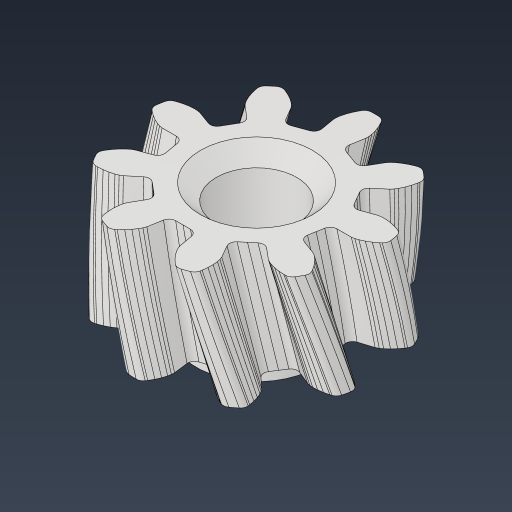
# Autodesk Inventor part: Planetengetriebe Planet
Saved by Autodesk Inventor 2023.1 (Build 271208000, 208)
## iProperties
Part Number: Planetengetriebe Planet
Material: Polyaryletherketon-Kunststoff
Document SubType Name: Modeling
Designer: rYan
Density: 1.32 g/cm^3
Appearance: Glatt - Weiß
Mass: 0.315298 g
Surface Area: 4.33242 cm^2
Volume: 0.238862 cm^3
Author: rYan
Autodesk Inventor part; units mm, degrees
ref_plane "YZ Plane" through (0, 0, 0) normal (1, 0, 0) x (0, 1, 0)
ref_plane "XZ Plane" through (0, 0, 0) normal (0, 1, 0) x (-1, 0, 0)
ref_plane "XY Plane" through (0, 0, 0) normal (0, 0, 1) x (1, 0, 0)
sketch "Skizze1" plane through (0, 0, 0) normal (0, 0, 1) x (1, 0, 0)
  circle A0 centre (0, 0) radius 3.3 construction
  circle A1 centre (0, 0) radius 4.2286 construction
  circle A2 centre (0, 0) radius 4.5 construction
  circle A3 centre (0, 0) radius 5.3 construction
  line L0 (0, 7.42) -> (0, -7.42) construction
  arc A4 (0.7096, 4.4437) -> (-0.7096, 4.4437) centre (0, 0) ccw
  arc A5 (0.729, 4.1653) -> (-0.729, 4.1653) centre (0, 0) ccw
  arc A6 (0.3429, 5.2889) -> (-0.3429, 5.2889) centre (0, 0) ccw
  line L1 (-0.729, 4.1653) -> (-0.6182, 3.5324)
  line L2 (0.729, 4.1653) -> (0.6182, 3.5324)
  arc A7 (0.6182, 3.5324) -> (0.8111, 3.1988) centre (0.9137, 3.4807) ccw
  arc A8 (-0.8111, 3.1988) -> (-0.6182, 3.5324) centre (-0.9137, 3.4807) ccw
  line L3 (0, 0) -> (1.1229, 3.0853)
  line L4 (0, 0) -> (-1.1229, 3.0853)
  line L5 (1.1229, 3.0853) -> (0.8111, 3.1988)
  line L6 (-0.8111, 3.1988) -> (-1.1229, 3.0853)
  arc A9 (0.5742, 4.8662) -> (-0.5742, 4.8662) centre (0, 0) ccw construction
  arc A10 (0.7294, 4.3029) -> (-0.7294, 4.3029) centre (0, 0) ccw construction
  arc A11 (0.4698, 5.0783) -> (-0.4698, 5.0783) centre (0, 0) ccw construction
  line L7 (0.3429, 5.2889) -> (0.4698, 5.0783)
  line L8 (0.4698, 5.0783) -> (0.5742, 4.8662)
  line L9 (0.7096, 4.4437) -> (0.7294, 4.3029)
  line L10 (0.7294, 4.3029) -> (0.729, 4.1653)
  arc A12 (0.655, 4.6541) -> (-0.655, 4.6541) centre (0, 0) ccw construction
  line L11 (0.5742, 4.8662) -> (0.655, 4.6541)
  line L12 (0.7096, 4.4437) -> (0.655, 4.6541)
  line L13 (-0.3429, 5.2889) -> (-0.4698, 5.0783)
  line L14 (-0.4698, 5.0783) -> (-0.5742, 4.8662)
  line L15 (-0.5742, 4.8662) -> (-0.655, 4.6541)
  line L16 (-0.655, 4.6541) -> (-0.7096, 4.4437)
  line L17 (-0.7096, 4.4437) -> (-0.7294, 4.3029)
  line L18 (-0.7294, 4.3029) -> (-0.729, 4.1653)
  dimension "d0" = 6.6
  dimension "d1" = 8.4572
  dimension "d2" = 9
  dimension "d3" = 10.6
  dimension "d4" = 1.4252
  dimension "d12" = 1.4653
  dimension "d13" = 0.6862
  dimension "d19" = 0.3
  dimension "d20" = 0.3
  dimension "d21" = 40
  dimension "d29" = 1.1511
  dimension "d30" = 4.9
  dimension "d31" = 4.3643
  dimension "d32" = 1.4657
  dimension "d33" = 5.1
  dimension "d34" = 0.9409
  dimension "d35" = 4.7
  dimension "d36" = 1.3142
  constraints: 36 end point, 26 point on circle, 13 centre point, 11 coincident, 7 symmetric about line, 4 tangent, 2 perpendicular, 2 point on line, 1 other
  measures "d0" diameter of A0
  measures "d1" diameter of A1
  measures "d2" diameter of A2
  measures "d3" diameter of A3
  measures "d19" radius of A7
  measures "d20" radius of A8
  measures "d21" angle of L3 L4
  measures "d30" radius of A9
  measures "d31" radius of A10
  measures "d33" radius of A11
  measures "d35" radius of A12
coil "Spirale2" sketch "Skizze1" operation add axis through (0, 0, -10) along (0, 0, -1) pitch 104.0668 turns 0.048046 hand left
fillet "Rundung2" radius 0.3 2 edges at (-1.1343, 5.1772, -2.5) (-0.4563, 5.2803, -2.5)
pattern_circular "Runde Anordnung4" count 9 over 360 about axis through (0, 0, -10) along (0, 0, 1) of "Spirale2", "Rundung2"
sketch "Skizze2" plane through (0, 0, 0) normal (0, 0, 1) x (1, 0, 0)
  point P0 (0, 0)
  point P1 (0, 0)
  constraints: 1 coincident
hole "Bohrung1" at (0, 0, 0) direction (0, 0, -1) diameter 3.6 end through all
sketch "Skizze4" plane through (-0.1031, 0.7973, -5) normal (0, 0, -1) x (-0.7537864, -0.6571196, 0)
  circle A0 centre (0.4462, -0.6688) radius 2.7
  circle A1 centre (0.4462, -0.6688) radius 1.8 projected
  dimension "d40" = 5.4
  constraints: 2 coincident, 1 centre point
  measures "d40" diameter of A0
extrude "Extrusion3" add sketch "Skizze4" along normal blind 0.8
chamfer "Fase1" distance 0.5 angle 45 1 edges at (1.3568, 1.1828, -5.8)
chamfer "Fase2" distance 0.7 angle 45 1 edges at (0, 1.8, 0)
sketch "Skizze10" plane through (-0.6182, 3.5324, 0) normal (0, 0, 1) x (0.9850278, 0.1723953, 0)
  arc A0 (1.0773, 1.6033) -> (0.7491, 1.6607) centre (0, -3.5861) ccw projected
  line L0 (0.4653, 1.5576) -> (0.4127, 1.4972) projected
  line L1 (0.4127, 1.4972) -> (0.2733, 1.3063) projected
  line L2 (0.2733, 1.3063) -> (0.1572, 1.1113) projected
  line L3 (0.1572, 1.1113) -> (0.0671, 0.9134) projected
  line L4 (0.0671, 0.9134) -> (0.0233, 0.7782) projected
  line L5 (0.0233, 0.7782) -> (0, 0.6425) projected
  line L6 (0, 0.6425) -> (0, 0) projected
  arc A1 (-0.2475, -0.2954) -> (0, 0) centre (-0.3, 0) ccw projected
  line L7 (-0.2475, -0.2954) -> (-0.5742, -0.3534) projected
  line L8 (-0.5742, -0.3534) -> (-0.901, -0.4115) projected
  arc A2 (-1.2351, -0.2194) -> (-0.901, -0.4115) centre (-0.9534, -0.1161) ccw projected
  line L9 (-1.2351, -0.2194) -> (-1.4564, 0.3838) projected
  line L10 (-1.4564, 0.3838) -> (-1.525, 0.5031) projected
  line L11 (-1.525, 0.5031) -> (-1.6126, 0.615) projected
  line L12 (-1.6126, 0.615) -> (-1.7654, 0.7698) projected
  line L13 (-1.7654, 0.7698) -> (-1.9415, 0.9129) projected
  line L14 (-1.9415, 0.9129) -> (-2.1382, 1.0441) projected
  line L15 (-2.1382, 1.0441) -> (-2.2084, 1.0827) projected
  arc A3 (-2.5104, 1.0817) -> (-2.7987, 0.9147) centre (0, -3.5861) ccw projected
  line L16 (-2.9499, 0.6533) -> (-2.9513, 0.5732) projected
  line L17 (-2.9513, 0.5732) -> (-2.9354, 0.3373) projected
  line L18 (-2.9354, 0.3373) -> (-2.899, 0.1134) projected
  line L19 (-2.899, 0.1134) -> (-2.8408, -0.0962) projected
  line L20 (-2.8408, -0.0962) -> (-2.7874, -0.2279) projected
  line L21 (-2.7874, -0.2279) -> (-2.7181, -0.3468) projected
  line L22 (-2.7181, -0.3468) -> (-2.3051, -0.839) projected
  arc A4 (-2.3048, -1.2244) -> (-2.3051, -0.839) centre (-2.5349, -1.0318) ccw projected
  line L23 (-2.3048, -1.2244) -> (-2.5178, -1.4788) projected
  line L24 (-2.5178, -1.4788) -> (-2.7308, -1.7333) projected
  arc A5 (-3.1102, -1.8009) -> (-2.7308, -1.7333) centre (-2.9608, -1.5408) ccw projected
  line L25 (-3.1102, -1.8009) -> (-3.6675, -1.4811) projected
  line L26 (-3.6675, -1.4811) -> (-3.7967, -1.4338) projected
  line L27 (-3.7967, -1.4338) -> (-3.9358, -1.4044) projected
  line L28 (-3.9358, -1.4044) -> (-4.1523, -1.3841) projected
  line L29 (-4.1523, -1.3841) -> (-4.3792, -1.3877) projected
  line L30 (-4.3792, -1.3877) -> (-4.6141, -1.4136) projected
  line L31 (-4.6141, -1.4136) -> (-4.6927, -1.4291) projected
  arc A6 (-4.9234, -1.624) -> (-5.037, -1.9372) centre (0, -3.5861) ccw projected
  line L32 (-4.9848, -2.2347) -> (-4.9344, -2.2969) projected
  line L33 (-4.9344, -2.2969) -> (-4.7706, -2.4674) projected
  line L34 (-4.7706, -2.4674) -> (-4.5987, -2.6156) projected
  line L35 (-4.5987, -2.6156) -> (-4.4195, -2.7387) projected
  line L36 (-4.4195, -2.7387) -> (-4.2939, -2.8053) projected
  line L37 (-4.2939, -2.8053) -> (-4.1644, -2.8518) projected
  line L38 (-4.1644, -2.8518) -> (-3.5316, -2.9634) projected
  arc A7 (-3.2837, -3.2584) -> (-3.5316, -2.9634) centre (-3.5837, -3.2588) ccw projected
  line L39 (-3.2837, -3.2584) -> (-3.2833, -3.5903) projected
  line L40 (-3.2833, -3.5903) -> (-3.2828, -3.9221) projected
  arc A8 (-3.53, -4.2178) -> (-3.2828, -3.9221) centre (-3.5828, -3.9225) ccw projected
  line L41 (-3.53, -4.2178) -> (-4.1625, -4.331) projected
  line L42 (-4.1625, -4.331) -> (-4.2919, -4.3778) projected
  line L43 (-4.2919, -4.3778) -> (-4.4173, -4.4447) projected
  line L44 (-4.4173, -4.4447) -> (-4.5962, -4.5683) projected
  line L45 (-4.5962, -4.5683) -> (-4.7677, -4.7169) projected
  line L46 (-4.7677, -4.7169) -> (-4.9311, -4.8878) projected
  line L47 (-4.9311, -4.8878) -> (-4.9813, -4.9502) projected
  arc A9 (-5.0328, -5.2478) -> (-4.9184, -5.5607) centre (0, -3.5861) ccw projected
  line L48 (-4.6872, -5.755) -> (-4.6086, -5.7703) projected
  line L49 (-4.6086, -5.7703) -> (-4.3736, -5.7956) projected
  line L50 (-4.3736, -5.7956) -> (-4.1466, -5.7986) projected
  line L51 (-4.1466, -5.7986) -> (-3.9302, -5.7777) projected
  line L52 (-3.9302, -5.7777) -> (-3.7912, -5.748) projected
  line L53 (-3.7912, -5.748) -> (-3.6621, -5.7004) projected
  line L54 (-3.6621, -5.7004) -> (-3.1056, -5.3791) projected
  arc A10 (-2.7261, -5.4458) -> (-3.1056, -5.3791) centre (-2.9556, -5.6389) ccw projected
  line L55 (-2.7261, -5.4458) -> (-2.5124, -5.6997) projected
  line L56 (-2.5124, -5.6997) -> (-2.2988, -5.9537) projected
  arc A11 (-2.2981, -6.339) -> (-2.2988, -5.9537) centre (-2.5284, -6.1468) ccw projected
  line L57 (-2.2981, -6.339) -> (-2.7099, -6.8323) projected
  line L58 (-2.7099, -6.8323) -> (-2.7789, -6.9514) projected
  line L59 (-2.7789, -6.9514) -> (-2.832, -7.0832) projected
  line L60 (-2.832, -7.0832) -> (-2.8896, -7.2929) projected
  line L61 (-2.8896, -7.2929) -> (-2.9254, -7.517) projected
  line L62 (-2.9254, -7.517) -> (-2.9407, -7.7529) projected
  line L63 (-2.9407, -7.7529) -> (-2.9391, -7.833) projected
  arc A12 (-2.7872, -8.094) -> (-2.4985, -8.2602) centre (0, -3.5861) ccw projected
  line L64 (-2.1965, -8.2605) -> (-2.1264, -8.2216) projected
  line L65 (-2.1264, -8.2216) -> (-1.9301, -8.0899) projected
  line L66 (-1.9301, -8.0899) -> (-1.7543, -7.9464) projected
  line L67 (-1.7543, -7.9464) -> (-1.6019, -7.7913) projected
  line L68 (-1.6019, -7.7913) -> (-1.5146, -7.6792) projected
  line L69 (-1.5146, -7.6792) -> (-1.4463, -7.5597) projected
  line L70 (-1.4463, -7.5597) -> (-1.2265, -6.9559) projected
  arc A13 (-0.8929, -6.763) -> (-1.2265, -6.9559) centre (-0.9446, -7.0585) ccw projected
  line L71 (-0.8929, -6.763) -> (-0.566, -6.8202) projected
  line L72 (-0.566, -6.8202) -> (-0.2392, -6.8774) projected
  arc A14 (0.0091, -7.1721) -> (-0.2392, -6.8774) centre (-0.2909, -7.1729) ccw projected
  line L73 (0.0091, -7.1721) -> (0.0108, -7.8147) projected
  line L74 (0.0108, -7.8147) -> (0.0344, -7.9503) projected
  line L75 (0.0344, -7.9503) -> (0.0785, -8.0854) projected
  line L76 (0.0785, -8.0854) -> (0.1692, -8.283) projected
  line L77 (0.1692, -8.283) -> (0.2857, -8.4777) projected
  line L78 (0.2857, -8.4777) -> (0.4256, -8.6683) projected
  line L79 (0.4256, -8.6683) -> (0.4784, -8.7286) projected
  arc A15 (0.7625, -8.8309) -> (1.0905, -8.7727) centre (0, -3.5861) ccw projected
  line L80 (1.322, -8.5787) -> (1.3508, -8.504) projected
  line L81 (1.3508, -8.504) -> (1.4165, -8.2769) projected
  line L82 (1.4165, -8.2769) -> (1.4589, -8.0539) projected
  line L83 (1.4589, -8.0539) -> (1.4759, -7.8372) projected
  line L84 (1.4759, -7.8372) -> (1.4707, -7.6951) projected
  line L85 (1.4707, -7.6951) -> (1.4463, -7.5597) projected
  line L86 (1.4463, -7.5597) -> (1.2265, -6.9559) projected
  arc A16 (1.3581, -6.5937) -> (1.2265, -6.9559) centre (1.5084, -6.8533) ccw projected
  line L87 (1.3581, -6.5937) -> (1.6453, -6.4274) projected
  line L88 (1.6453, -6.4274) -> (1.9324, -6.2611) projected
  arc A17 (2.3121, -6.3273) -> (1.9324, -6.2611) centre (2.0827, -6.5207) ccw projected
  line L89 (2.3121, -6.3273) -> (2.7263, -6.8185) projected
  line L90 (2.7263, -6.8185) -> (2.8316, -6.9071) projected
  line L91 (2.8316, -6.9071) -> (2.9522, -6.9823) projected
  line L92 (2.9522, -6.9823) -> (3.1487, -7.0754) projected
  line L93 (3.1487, -7.0754) -> (3.3632, -7.1497) projected
  line L94 (3.3632, -7.1497) -> (3.5928, -7.2057) projected
  line L95 (3.5928, -7.2057) -> (3.672, -7.218) projected
  arc A18 (3.9554, -7.1138) -> (4.1693, -6.8583) centre (0, -3.5861) ccw projected
  line L96 (4.222, -6.5609) -> (4.1959, -6.4851) projected
  line L97 (4.1959, -6.4851) -> (4.1003, -6.2689) projected
  line L98 (4.1003, -6.2689) -> (3.9894, -6.0709) projected
  line L99 (3.9894, -6.0709) -> (3.8631, -5.8939) projected
  line L100 (3.8631, -5.8939) -> (3.7679, -5.7884) projected
  line L101 (3.7679, -5.7884) -> (3.6621, -5.7004) projected
  line L102 (3.6621, -5.7004) -> (3.1056, -5.3791) projected
  arc A19 (2.9736, -5.0171) -> (3.1056, -5.3791) centre (3.2556, -5.1193) ccw projected
  line L103 (2.9736, -5.0171) -> (3.0867, -4.7051) projected
  line L104 (3.0867, -4.7051) -> (3.1998, -4.3931) projected
  arc A20 (3.5332, -4.1998) -> (3.1998, -4.3931) centre (3.4818, -4.4954) ccw projected
  line L105 (3.5332, -4.1998) -> (4.1662, -4.3098) projected
  line L106 (4.1662, -4.3098) -> (4.3038, -4.31) projected
  line L107 (4.3038, -4.31) -> (4.4446, -4.2901) projected
  line L108 (4.4446, -4.2901) -> (4.655, -4.2351) projected
  line L109 (4.655, -4.2351) -> (4.867, -4.1541) projected
  line L110 (4.867, -4.1541) -> (5.0789, -4.0494) projected
  line L111 (5.0789, -4.0494) -> (5.1475, -4.008) projected
  arc A21 (5.2976, -3.7459) -> (5.2972, -3.4128) centre (0, -3.5861) ccw projected
  line L112 (5.1464, -3.1511) -> (5.0777, -3.1098) projected
  line L113 (5.0777, -3.1098) -> (4.8655, -3.0056) projected
  line L114 (4.8655, -3.0056) -> (4.6533, -2.9252) projected
  line L115 (4.6533, -2.9252) -> (4.4428, -2.8708) projected
  line L116 (4.4428, -2.8708) -> (4.302, -2.8512) projected
  line L117 (4.302, -2.8512) -> (4.1644, -2.8518) projected
  line L118 (4.1644, -2.8518) -> (3.5316, -2.9634) projected
  arc A22 (3.1977, -2.7709) -> (3.5316, -2.9634) centre (3.4795, -2.6679) ccw projected
  line L119 (3.1977, -2.7709) -> (3.0838, -2.4592) projected
  line L120 (3.0838, -2.4592) -> (2.9699, -2.1475) projected
  arc A23 (3.1011, -1.7851) -> (2.9699, -2.1475) centre (3.2517, -2.0446) ccw projected
  line L121 (3.1011, -1.7851) -> (3.6567, -1.4625) projected
  line L122 (3.6567, -1.4625) -> (3.7623, -1.3742) projected
  line L123 (3.7623, -1.3742) -> (3.8573, -1.2684) projected
  line L124 (3.8573, -1.2684) -> (3.9831, -1.0911) projected
  line L125 (3.9831, -1.0911) -> (4.0934, -0.8928) projected
  line L126 (4.0934, -0.8928) -> (4.1885, -0.6764) projected
  line L127 (4.1885, -0.6764) -> (4.2144, -0.6005) projected
  arc A24 (4.1609, -0.3033) -> (3.9465, -0.0483) centre (0, -3.5861) ccw projected
  line L128 (3.6627, 0.0552) -> (3.5836, 0.0426) projected
  line L129 (3.5836, 0.0426) -> (3.3541, -0.014) projected
  line L130 (3.3541, -0.014) -> (3.1398, -0.0887) projected
  line L131 (3.1398, -0.0887) -> (2.9436, -0.1824) projected
  line L132 (2.9436, -0.1824) -> (2.8231, -0.2579) projected
  line L133 (2.8231, -0.2579) -> (2.7181, -0.3468) projected
  line L134 (2.7181, -0.3468) -> (2.3051, -0.839) projected
  arc A25 (1.9256, -0.9061) -> (2.3051, -0.839) centre (2.0753, -0.6461) ccw projected
  line L135 (1.9256, -0.9061) -> (1.638, -0.7406) projected
  line L136 (1.638, -0.7406) -> (1.3504, -0.575) projected
  arc A26 (1.2179, -0.2132) -> (1.3504, -0.575) centre (1.5001, -0.315) ccw projected
  line L137 (1.2179, -0.2132) -> (1.4362, 0.3912) projected
  line L138 (1.4362, 0.3912) -> (1.4603, 0.5267) projected
  line L139 (1.4603, 0.5267) -> (1.4651, 0.6687) projected
  line L140 (1.4651, 0.6687) -> (1.4475, 0.8855) projected
  line L141 (1.4475, 0.8855) -> (1.4046, 1.1083) projected
  line L142 (1.4046, 1.1083) -> (1.3382, 1.3352) projected
  line L143 (1.3382, 1.3352) -> (1.3093, 1.4099) projected
  circle A27 centre (0, -3.5861) radius 2.5 projected
  line L144 (3.632, -7.0094) -> (3.4197, -6.9576)
  line L145 (3.4197, -6.9576) -> (3.2245, -6.89)
  line L146 (3.2245, -6.89) -> (3.0483, -6.8065)
  line L147 (3.0483, -6.8065) -> (2.9495, -6.7449)
  line L148 (2.9495, -6.7449) -> (2.8682, -6.6765)
  line L149 (2.8682, -6.6765) -> (2.465, -6.1984)
  arc A28 (2.465, -6.1984) -> (1.8322, -6.088) centre (2.0827, -6.5207) ccw
  line L150 (1.8322, -6.088) -> (1.545, -6.2543)
  line L151 (1.545, -6.2543) -> (1.2579, -6.4206)
  arc A29 (1.2579, -6.4206) -> (1.0386, -7.0243) centre (1.5084, -6.8533) ccw
  line L152 (1.0386, -7.0243) -> (1.2525, -7.612)
  line L153 (1.2525, -7.612) -> (1.2714, -7.7166)
  line L154 (1.2714, -7.7166) -> (1.2756, -7.8329)
  line L155 (1.2756, -7.8329) -> (1.2603, -8.0274)
  line L156 (1.2603, -8.0274) -> (1.2218, -8.2303)
  line L157 (1.2218, -8.2303) -> (1.161, -8.4402)
  line L158 (1.161, -8.4402) -> (1.1353, -8.507)
  arc A30 (0.7337, -8.633) -> (1.0494, -8.5769) centre (0, -3.5861) ccw
  line L159 (0.629, -8.597) -> (0.5818, -8.5431)
  line L160 (0.5818, -8.5431) -> (0.4525, -8.3669)
  line L161 (0.4525, -8.3669) -> (0.3464, -8.1897)
  line L162 (0.3464, -8.1897) -> (0.2651, -8.0125)
  line L163 (0.2651, -8.0125) -> (0.229, -7.9018)
  line L164 (0.229, -7.9018) -> (0.2107, -7.7971)
  line L165 (0.2107, -7.7971) -> (0.2091, -7.1716)
  arc A31 (0.2091, -7.1716) -> (-0.2047, -6.6804) centre (-0.2909, -7.1729) ccw
  line L166 (-0.2047, -6.6804) -> (-0.5315, -6.6232)
  line L167 (-0.5315, -6.6232) -> (-0.8584, -6.566)
  arc A32 (-0.8584, -6.566) -> (-1.4144, -6.8875) centre (-0.9446, -7.0585) ccw
  line L168 (-1.4144, -6.8875) -> (-1.6284, -7.4752)
  line L169 (-1.6284, -7.4752) -> (-1.6811, -7.5675)
  line L170 (-1.6811, -7.5675) -> (-1.7527, -7.6593)
  line L171 (-1.7527, -7.6593) -> (-1.8893, -7.7984)
  line L172 (-1.8893, -7.7984) -> (-2.0493, -7.9291)
  line L173 (-2.0493, -7.9291) -> (-2.2308, -8.0508)
  line L174 (-2.2308, -8.0508) -> (-2.2934, -8.0855)
  arc A33 (-2.6821, -7.9239) -> (-2.4042, -8.0838) centre (0, -3.5861) ccw
  line L175 (-2.7391, -7.8289) -> (-2.7406, -7.7573)
  line L176 (-2.7406, -7.7573) -> (-2.7265, -7.5393)
  line L177 (-2.7265, -7.5393) -> (-2.6938, -7.3353)
  line L178 (-2.6938, -7.3353) -> (-2.6421, -7.1473)
  line L179 (-2.6421, -7.1473) -> (-2.5987, -7.0393)
  line L180 (-2.5987, -7.0393) -> (-2.5454, -6.9474)
  line L181 (-2.5454, -6.9474) -> (-2.1446, -6.4672)
  arc A34 (-2.1446, -6.4672) -> (-2.1458, -5.8249) centre (-2.5284, -6.1468) ccw
  line L182 (-2.1458, -5.8249) -> (-2.3594, -5.571)
  line L183 (-2.3594, -5.571) -> (-2.573, -5.317)
  arc A35 (-2.573, -5.317) -> (-3.2056, -5.2059) centre (-2.9556, -5.6389) ccw
  line L184 (-3.2056, -5.2059) -> (-3.7473, -5.5186)
  line L185 (-3.7473, -5.5186) -> (-3.847, -5.5554)
  line L186 (-3.847, -5.5554) -> (-3.9608, -5.5798)
  line L187 (-3.9608, -5.5798) -> (-4.1549, -5.5985)
  line L188 (-4.1549, -5.5985) -> (-4.3615, -5.5958)
  line L189 (-4.3615, -5.5958) -> (-4.5787, -5.5724)
  line L190 (-4.5787, -5.5724) -> (-4.6491, -5.5587)
  arc A36 (-4.8429, -5.185) -> (-4.7328, -5.4862) centre (0, -3.5861) ccw
  line L191 (-4.8256, -5.0756) -> (-4.7806, -5.0198)
  line L192 (-4.7806, -5.0198) -> (-4.6297, -4.8619)
  line L193 (-4.6297, -4.8619) -> (-4.4735, -4.7266)
  line L194 (-4.4735, -4.7266) -> (-4.3131, -4.6158)
  line L195 (-4.3131, -4.6158) -> (-4.2104, -4.561)
  line L196 (-4.2104, -4.561) -> (-4.1105, -4.5248)
  line L197 (-4.1105, -4.5248) -> (-3.4948, -4.4147)
  arc A37 (-3.4948, -4.4147) -> (-3.0828, -3.9218) centre (-3.5828, -3.9225) ccw
  line L198 (-3.0828, -3.9218) -> (-3.0833, -3.59)
  line L199 (-3.0833, -3.59) -> (-3.0837, -3.2582)
  arc A38 (-3.0837, -3.2582) -> (-3.4969, -2.7664) centre (-3.5837, -3.2588) ccw
  line L200 (-3.4969, -2.7664) -> (-4.1128, -2.6578)
  line L201 (-4.1128, -2.6578) -> (-4.2129, -2.6219)
  line L202 (-4.2129, -2.6219) -> (-4.3157, -2.5674)
  line L203 (-4.3157, -2.5674) -> (-4.4764, -2.4569)
  line L204 (-4.4764, -2.4569) -> (-4.6329, -2.3221)
  line L205 (-4.6329, -2.3221) -> (-4.7843, -2.1645)
  line L206 (-4.7843, -2.1645) -> (-4.8293, -2.1088)
  arc A39 (-4.7376, -1.698) -> (-4.8469, -1.9994) centre (0, -3.5861) ccw
  line L207 (-4.6541, -1.6253) -> (-4.5838, -1.6115)
  line L208 (-4.5838, -1.6115) -> (-4.3666, -1.5875)
  line L209 (-4.3666, -1.5875) -> (-4.16, -1.5842)
  line L210 (-4.16, -1.5842) -> (-3.9659, -1.6025)
  line L211 (-3.9659, -1.6025) -> (-3.852, -1.6265)
  line L212 (-3.852, -1.6265) -> (-3.7522, -1.663)
  line L213 (-3.7522, -1.663) -> (-3.2097, -1.9744)
  arc A40 (-3.2097, -1.9744) -> (-2.5774, -1.8617) centre (-2.9608, -1.5408) ccw
  line L214 (-2.5774, -1.8617) -> (-2.3644, -1.6072)
  line L215 (-2.3644, -1.6072) -> (-2.1515, -1.3527)
  arc A41 (-2.1515, -1.3527) -> (-2.1519, -0.7104) centre (-2.5349, -1.0318) ccw
  line L216 (-2.1519, -0.7104) -> (-2.5539, -0.2313)
  line L217 (-2.5539, -0.2313) -> (-2.6075, -0.1395)
  line L218 (-2.6075, -0.1395) -> (-2.6512, -0.0316)
  line L219 (-2.6512, -0.0316) -> (-2.7033, 0.1563)
  line L220 (-2.7033, 0.1563) -> (-2.7365, 0.3602)
  line L221 (-2.7365, 0.3602) -> (-2.7512, 0.5782)
  line L222 (-2.7512, 0.5782) -> (-2.7499, 0.6498)
  arc A42 (-2.4156, 0.9056) -> (-2.6931, 0.7449) centre (0, -3.5861) ccw
  line L223 (-2.3049, 0.9075) -> (-2.2421, 0.873)
  line L224 (-2.2421, 0.873) -> (-2.0603, 0.7517)
  line L225 (-2.0603, 0.7517) -> (-1.9, 0.6214)
  line L226 (-1.9, 0.6214) -> (-1.763, 0.4827)
  line L227 (-1.763, 0.4827) -> (-1.6912, 0.391)
  line L228 (-1.6912, 0.391) -> (-1.6383, 0.2989)
  line L229 (-1.6383, 0.2989) -> (-1.4228, -0.2883)
  arc A43 (-1.4228, -0.2883) -> (-0.866, -0.6084) centre (-0.9534, -0.1161) ccw
  line L230 (-0.866, -0.6084) -> (-0.5393, -0.5503)
  line L231 (-0.5393, -0.5503) -> (-0.2125, -0.4923)
  arc A44 (-0.2125, -0.4923) -> (0.2, 0) centre (-0.3, 0) ccw
  line L232 (0.2, 0) -> (0.2, 0.6255)
  line L233 (0.2, 0.6255) -> (0.218, 0.7302)
  line L234 (0.218, 0.7302) -> (0.2538, 0.841)
  line L235 (0.2538, 0.841) -> (0.3347, 1.0184)
  line L236 (0.3347, 1.0184) -> (0.4403, 1.1959)
  line L237 (0.4403, 1.1959) -> (0.5692, 1.3724)
  line L238 (0.5692, 1.3724) -> (0.6162, 1.4264)
  arc A45 (1.0367, 1.4074) -> (0.7209, 1.4627) centre (0, -3.5861) ccw
  line L239 (1.1228, 1.3378) -> (1.1487, 1.271)
  line L240 (1.1487, 1.271) -> (1.21, 1.0612)
  line L241 (1.21, 1.0612) -> (1.249, 0.8584)
  line L242 (1.249, 0.8584) -> (1.2648, 0.664)
  line L243 (1.2648, 0.664) -> (1.2609, 0.5477)
  line L244 (1.2609, 0.5477) -> (1.2422, 0.4431)
  line L245 (1.2422, 0.4431) -> (1.0298, -0.1452)
  arc A46 (1.0298, -0.1452) -> (1.2507, -0.7484) centre (1.5001, -0.315) ccw
  line L246 (1.2507, -0.7484) -> (1.5382, -0.9139)
  line L247 (1.5382, -0.9139) -> (1.8258, -1.0795)
  arc A47 (1.8258, -1.0795) -> (2.4583, -0.9675) centre (2.0753, -0.6461) ccw
  line L248 (2.4583, -0.9675) -> (2.8603, -0.4884)
  line L249 (2.8603, -0.4884) -> (2.9415, -0.4197)
  line L250 (2.9415, -0.4197) -> (3.0401, -0.3579)
  line L251 (3.0401, -0.3579) -> (3.2161, -0.274)
  line L252 (3.2161, -0.274) -> (3.4111, -0.2059)
  line L253 (3.4111, -0.2059) -> (3.6233, -0.1536)
  line L254 (3.6233, -0.1536) -> (3.694, -0.1424)
  arc A48 (4.0039, -0.4272) -> (3.7975, -0.1818) centre (0, -3.5861) ccw
  line L255 (4.0251, -0.5359) -> (4.002, -0.6037)
  line L256 (4.002, -0.6037) -> (3.9141, -0.8038)
  line L257 (3.9141, -0.8038) -> (3.8137, -0.9843)
  line L258 (3.8137, -0.9843) -> (3.7008, -1.1433)
  line L259 (3.7008, -1.1433) -> (3.623, -1.2299)
  line L260 (3.623, -1.2299) -> (3.5415, -1.2981)
  line L261 (3.5415, -1.2981) -> (3.0006, -1.6122)
  arc A49 (3.0006, -1.6122) -> (2.7821, -2.2162) centre (3.2517, -2.0446) ccw
  line L262 (2.7821, -2.2162) -> (2.896, -2.5279)
  line L263 (2.896, -2.5279) -> (3.0099, -2.8395)
  arc A50 (3.0099, -2.8395) -> (3.5663, -3.1603) centre (3.4795, -2.6679) ccw
  line L264 (3.5663, -3.1603) -> (4.1823, -3.0517)
  line L265 (4.1823, -3.0517) -> (4.2886, -3.0513)
  line L266 (4.2886, -3.0513) -> (4.4039, -3.0673)
  line L267 (4.4039, -3.0673) -> (4.5927, -3.1161)
  line L268 (4.5927, -3.1161) -> (4.7858, -3.1893)
  line L269 (4.7858, -3.1893) -> (4.982, -3.2856)
  line L270 (4.982, -3.2856) -> (5.0434, -3.3225)
  arc A51 (5.0977, -3.7399) -> (5.0973, -3.4193) centre (0, -3.5861) ccw
  line L271 (5.044, -3.8368) -> (4.9827, -3.8739)
  line L272 (4.9827, -3.8739) -> (4.7868, -3.9707)
  line L273 (4.7868, -3.9707) -> (4.5938, -4.0444)
  line L274 (4.5938, -4.0444) -> (4.4052, -4.0936)
  line L275 (4.4052, -4.0936) -> (4.2899, -4.11)
  line L276 (4.2899, -4.11) -> (4.1836, -4.1098)
  line L277 (4.1836, -4.1098) -> (3.5674, -4.0028)
  arc A52 (3.5674, -4.0028) -> (3.0118, -4.325) centre (3.4818, -4.4954) ccw
  line L278 (3.0118, -4.325) -> (2.8987, -4.6369)
  line L279 (2.8987, -4.6369) -> (2.7856, -4.9489)
  arc A53 (2.7856, -4.9489) -> (3.0056, -5.5523) centre (3.2556, -5.1193) ccw
  line L280 (3.0056, -5.5523) -> (3.5473, -5.8651)
  line L281 (3.5473, -5.8651) -> (3.629, -5.933)
  line L282 (3.629, -5.933) -> (3.707, -6.0194)
  line L283 (3.707, -6.0194) -> (3.8203, -6.1782)
  line L284 (3.8203, -6.1782) -> (3.9212, -6.3584)
  line L285 (3.9212, -6.3584) -> (4.0095, -6.5583)
  line L286 (4.0095, -6.5583) -> (4.0328, -6.626)
  arc A54 (3.8062, -6.9806) -> (4.0119, -6.7348) centre (0, -3.5861) ccw
  line L287 (3.7028, -7.0204) -> (3.632, -7.0094)
  line L288 (3.6412, -7.4156) -> (3.5537, -7.402)
  line L289 (3.5537, -7.402) -> (3.3066, -7.3417)
  line L290 (3.3066, -7.3417) -> (3.0729, -7.2608)
  line L291 (3.0729, -7.2608) -> (2.8562, -7.1581)
  line L292 (2.8562, -7.1581) -> (2.7137, -7.0693)
  line L293 (2.7137, -7.0693) -> (2.5845, -6.9605)
  line L294 (2.5845, -6.9605) -> (2.1592, -6.4562)
  arc A55 (2.1592, -6.4562) -> (2.0326, -6.4342) centre (2.0827, -6.5207) ccw
  line L295 (2.0326, -6.4342) -> (1.7455, -6.6005)
  line L296 (1.7455, -6.6005) -> (1.4583, -6.7667)
  arc A56 (1.4583, -6.7667) -> (1.4144, -6.8875) centre (1.5084, -6.8533) ccw
  line L297 (1.4144, -6.8875) -> (1.64, -7.5073)
  line L298 (1.64, -7.5073) -> (1.6701, -7.6736)
  line L299 (1.6701, -7.6736) -> (1.6762, -7.8414)
  line L300 (1.6762, -7.8414) -> (1.6574, -8.0805)
  line L301 (1.6574, -8.0805) -> (1.6112, -8.3235)
  line L302 (1.6112, -8.3235) -> (1.5405, -8.5677)
  line L303 (1.5405, -8.5677) -> (1.5088, -8.6504)
  arc A57 (0.7913, -9.0289) -> (1.1317, -8.9684) centre (0, -3.5861) ccw
  line L304 (0.3278, -8.8602) -> (0.2695, -8.7935)
  line L305 (0.2695, -8.7935) -> (0.1189, -8.5885)
  line L306 (0.1189, -8.5885) -> (-0.0081, -8.3764)
  line L307 (-0.0081, -8.3764) -> (-0.1081, -8.1583)
  line L308 (-0.1081, -8.1583) -> (-0.1601, -7.9987)
  line L309 (-0.1601, -7.9987) -> (-0.1892, -7.8323)
  line L310 (-0.1892, -7.8323) -> (-0.1909, -7.1727)
  arc A58 (-0.1909, -7.1727) -> (-0.2736, -7.0744) centre (-0.2909, -7.1729) ccw
  line L311 (-0.2736, -7.0744) -> (-0.6005, -7.0172)
  line L312 (-0.6005, -7.0172) -> (-0.9274, -6.96)
  arc A59 (-0.9274, -6.96) -> (-1.0386, -7.0243) centre (-0.9446, -7.0585) ccw
  line L313 (-1.0386, -7.0243) -> (-1.2642, -7.6441)
  line L314 (-1.2642, -7.6441) -> (-1.348, -7.7908)
  line L315 (-1.348, -7.7908) -> (-1.4512, -7.9233)
  line L316 (-1.4512, -7.9233) -> (-1.6193, -8.0944)
  line L317 (-1.6193, -8.0944) -> (-1.8109, -8.2508)
  line L318 (-1.8109, -8.2508) -> (-2.022, -8.3925)
  line L319 (-2.022, -8.3925) -> (-2.0995, -8.4354)
  arc A60 (-2.8924, -8.2641) -> (-2.5928, -8.4366) centre (0, -3.5861) ccw
  line L320 (-3.1391, -7.837) -> (-3.1408, -7.7484)
  line L321 (-3.1408, -7.7484) -> (-3.1244, -7.4946)
  line L322 (-3.1244, -7.4946) -> (-3.0853, -7.2505)
  line L323 (-3.0853, -7.2505) -> (-3.0218, -7.0192)
  line L324 (-3.0218, -7.0192) -> (-2.9591, -6.8634)
  line L325 (-2.9591, -6.8634) -> (-2.8743, -6.7172)
  line L326 (-2.8743, -6.7172) -> (-2.4516, -6.2109)
  arc A61 (-2.4516, -6.2109) -> (-2.4519, -6.0824) centre (-2.5284, -6.1468) ccw
  line L327 (-2.4519, -6.0824) -> (-2.6655, -5.8285)
  line L328 (-2.6655, -5.8285) -> (-2.8791, -5.5746)
  arc A62 (-2.8791, -5.5746) -> (-3.0056, -5.5523) centre (-2.9556, -5.6389) ccw
  line L329 (-3.0056, -5.5523) -> (-3.5769, -5.8821)
  line L330 (-3.5769, -5.8821) -> (-3.7354, -5.9406)
  line L331 (-3.7354, -5.9406) -> (-3.8996, -5.9757)
  line L332 (-3.8996, -5.9757) -> (-4.1383, -5.9987)
  line L333 (-4.1383, -5.9987) -> (-4.3856, -5.9955)
  line L334 (-4.3856, -5.9955) -> (-4.6385, -5.9682)
  line L335 (-4.6385, -5.9682) -> (-4.7254, -5.9513)
  arc A63 (-5.2227, -5.3105) -> (-5.104, -5.6352) centre (0, -3.5861) ccw
  line L336 (-5.1371, -4.8247) -> (-5.0815, -4.7557)
  line L337 (-5.0815, -4.7557) -> (-4.9058, -4.5719)
  line L338 (-4.9058, -4.5719) -> (-4.7189, -4.41)
  line L339 (-4.7189, -4.41) -> (-4.5216, -4.2736)
  line L340 (-4.5216, -4.2736) -> (-4.3734, -4.1946)
  line L341 (-4.3734, -4.1946) -> (-4.2145, -4.1371)
  line L342 (-4.2145, -4.1371) -> (-3.5652, -4.0209)
  arc A64 (-3.5652, -4.0209) -> (-3.4828, -3.9223) centre (-3.5828, -3.9225) ccw
  line L343 (-3.4828, -3.9223) -> (-3.4833, -3.5905)
  line L344 (-3.4833, -3.5905) -> (-3.4837, -3.2587)
  arc A65 (-3.4837, -3.2587) -> (-3.5663, -3.1603) centre (-3.5837, -3.2588) ccw
  line L345 (-3.5663, -3.1603) -> (-4.2159, -3.0458)
  line L346 (-4.2159, -3.0458) -> (-4.3749, -2.9887)
  line L347 (-4.3749, -2.9887) -> (-4.5233, -2.91)
  line L348 (-4.5233, -2.91) -> (-4.721, -2.7742)
  line L349 (-4.721, -2.7742) -> (-4.9083, -2.6128)
  line L350 (-4.9083, -2.6128) -> (-5.0845, -2.4294)
  line L351 (-5.0845, -2.4294) -> (-5.1402, -2.3605)
  arc A66 (-5.1092, -1.5499) -> (-5.2271, -1.875) centre (0, -3.5861) ccw
  line L352 (-4.7314, -1.2329) -> (-4.6445, -1.2157)
  line L353 (-4.6445, -1.2157) -> (-4.3917, -1.1879)
  line L354 (-4.3917, -1.1879) -> (-4.1445, -1.1839)
  line L355 (-4.1445, -1.1839) -> (-3.9057, -1.2064)
  line L356 (-3.9057, -1.2064) -> (-3.7414, -1.2411)
  line L357 (-3.7414, -1.2411) -> (-3.5827, -1.2991)
  line L358 (-3.5827, -1.2991) -> (-3.0106, -1.6275)
  arc A67 (-3.0106, -1.6275) -> (-2.8842, -1.6049) centre (-2.9608, -1.5408) ccw
  line L359 (-2.8842, -1.6049) -> (-2.6712, -1.3505)
  line L360 (-2.6712, -1.3505) -> (-2.4582, -1.096)
  arc A68 (-2.4582, -1.096) -> (-2.4583, -0.9675) centre (-2.5349, -1.0318) ccw
  line L361 (-2.4583, -0.9675) -> (-2.8823, -0.4623)
  line L362 (-2.8823, -0.4623) -> (-2.9674, -0.3163)
  line L363 (-2.9674, -0.3163) -> (-3.0305, -0.1607)
  line L364 (-3.0305, -0.1607) -> (-3.0946, 0.0704)
  line L365 (-3.0946, 0.0704) -> (-3.1343, 0.3145)
  line L366 (-3.1343, 0.3145) -> (-3.1514, 0.5682)
  line L367 (-3.1514, 0.5682) -> (-3.1499, 0.6568)
  arc A69 (-2.6051, 1.2578) -> (-2.9043, 1.0846) centre (0, -3.5861) ccw
  line L368 (-2.1119, 1.2579) -> (-2.0343, 1.2151)
  line L369 (-2.0343, 1.2151) -> (-1.8227, 1.074)
  line L370 (-1.8227, 1.074) -> (-1.6308, 0.9181)
  line L371 (-1.6308, 0.9181) -> (-1.4623, 0.7474)
  line L372 (-1.4623, 0.7474) -> (-1.3587, 0.6152)
  line L373 (-1.3587, 0.6152) -> (-1.2745, 0.4687)
  line L374 (-1.2745, 0.4687) -> (-1.0473, -0.1505)
  arc A70 (-1.0473, -0.1505) -> (-0.9359, -0.2145) centre (-0.9534, -0.1161) ccw
  line L375 (-0.9359, -0.2145) -> (-0.6092, -0.1565)
  line L376 (-0.6092, -0.1565) -> (-0.2825, -0.0985)
  arc A71 (-0.2825, -0.0985) -> (-0.2, 0) centre (-0.3, 0) ccw
  line L377 (-0.2, 0) -> (-0.2, 0.6596)
  line L378 (-0.2, 0.6596) -> (-0.1714, 0.8261)
  line L379 (-0.1714, 0.8261) -> (-0.1197, 0.9859)
  line L380 (-0.1197, 0.9859) -> (-0.0203, 1.2042)
  line L381 (-0.0203, 1.2042) -> (0.1062, 1.4167)
  line L382 (0.1062, 1.4167) -> (0.2562, 1.622)
  line L383 (0.2562, 1.622) -> (0.3143, 1.6889)
  arc A72 (1.118, 1.7991) -> (0.7774, 1.8587) centre (0, -3.5861) ccw
  line L384 (1.4959, 1.4821) -> (1.5278, 1.3995)
  line L385 (1.5278, 1.3995) -> (1.5992, 1.1554)
  line L386 (1.5992, 1.1554) -> (1.646, 0.9126)
  line L387 (1.646, 0.9126) -> (1.6653, 0.6735)
  line L388 (1.6653, 0.6735) -> (1.6597, 0.5057)
  line L389 (1.6597, 0.5057) -> (1.6301, 0.3393)
  line L390 (1.6301, 0.3393) -> (1.406, -0.2811)
  arc A73 (1.406, -0.2811) -> (1.4502, -0.4017) centre (1.5001, -0.315) ccw
  line L391 (1.4502, -0.4017) -> (1.7378, -0.5673)
  line L392 (1.7378, -0.5673) -> (2.0254, -0.7328)
  arc A74 (2.0254, -0.7328) -> (2.1519, -0.7104) centre (2.0753, -0.6461) ccw
  line L393 (2.1519, -0.7104) -> (2.5759, -0.2051)
  line L394 (2.5759, -0.2051) -> (2.7048, -0.096)
  line L395 (2.7048, -0.096) -> (2.8471, -0.0068)
  line L396 (2.8471, -0.0068) -> (3.0636, 0.0965)
  line L397 (3.0636, 0.0965) -> (3.2971, 0.178)
  line L398 (3.2971, 0.178) -> (3.544, 0.2389)
  line L399 (3.544, 0.2389) -> (3.6315, 0.2527)
  arc A75 (4.318, -0.1794) -> (4.0954, 0.0851) centre (0, -3.5861) ccw
  line L400 (4.4037, -0.6652) -> (4.375, -0.749)
  line L401 (4.375, -0.749) -> (4.2728, -0.9818)
  line L402 (4.2728, -0.9818) -> (4.1525, -1.1979)
  line L403 (4.1525, -1.1979) -> (4.0137, -1.3935)
  line L404 (4.0137, -1.3935) -> (3.9015, -1.5185)
  line L405 (3.9015, -1.5185) -> (3.7719, -1.6268)
  line L406 (3.7719, -1.6268) -> (3.2015, -1.9581)
  arc A76 (3.2015, -1.9581) -> (3.1578, -2.0789) centre (3.2517, -2.0446) ccw
  line L407 (3.1578, -2.0789) -> (3.2717, -2.3906)
  line L408 (3.2717, -2.3906) -> (3.3856, -2.7022)
  arc A77 (3.3856, -2.7022) -> (3.4969, -2.7664) centre (3.4795, -2.6679) ccw
  line L409 (3.4969, -2.7664) -> (4.1465, -2.6519)
  line L410 (4.1465, -2.6519) -> (4.3154, -2.6511)
  line L411 (4.3154, -2.6511) -> (4.4817, -2.6743)
  line L412 (4.4817, -2.6743) -> (4.714, -2.7343)
  line L413 (4.714, -2.7343) -> (4.9452, -2.822)
  line L414 (4.9452, -2.822) -> (5.1735, -2.934)
  line L415 (5.1735, -2.934) -> (5.2494, -2.9797)
  arc A78 (5.4975, -3.752) -> (5.4971, -3.4062) centre (0, -3.5861) ccw
  line L416 (5.2509, -4.1791) -> (5.1751, -4.225)
  line L417 (5.1751, -4.225) -> (4.9471, -4.3376)
  line L418 (4.9471, -4.3376) -> (4.7161, -4.4259)
  line L419 (4.7161, -4.4259) -> (4.484, -4.4865)
  line L420 (4.484, -4.4865) -> (4.3178, -4.51)
  line L421 (4.3178, -4.51) -> (4.1488, -4.5097)
  line L422 (4.1488, -4.5097) -> (3.4989, -4.3969)
  arc A79 (3.4989, -4.3969) -> (3.3878, -4.4613) centre (3.4818, -4.4954) ccw
  line L423 (3.3878, -4.4613) -> (3.2747, -4.7733)
  line L424 (3.2747, -4.7733) -> (3.1616, -5.0852)
  arc A80 (3.1616, -5.0852) -> (3.2056, -5.2059) centre (3.2556, -5.1193) ccw
  line L425 (3.2056, -5.2059) -> (3.7769, -5.5357)
  line L426 (3.7769, -5.5357) -> (3.9068, -5.6438)
  line L427 (3.9068, -5.6438) -> (4.0193, -5.7684)
  line L428 (4.0193, -5.7684) -> (4.1586, -5.9637)
  line L429 (4.1586, -5.9637) -> (4.2794, -6.1794)
  line L430 (4.2794, -6.1794) -> (4.3822, -6.412)
  line L431 (4.3822, -6.412) -> (4.4111, -6.4958)
  arc A81 (4.1047, -7.2469) -> (4.3266, -6.9817) centre (0, -3.5861) ccw
  dimension "d94" = 0.2
  dimension "a_0_deg" = 20
  dimension "d91" = 0.2
  constraints: 576 end point, 108 point on circle, 54 centre point, 36 concentric, 35 parallel, 431 other
  measures "d91" distance between parallel lines of L94 L144
sketch "Skizze9" plane through (-0.6182, 3.5324, 0) normal (0, 0, 1) x (0.9850278, 0.1723953, 0)
  circle A0 centre (0, -3.5861) radius 5.2
  circle A1 centre (0, -3.5861) radius 7.2
  circle A2 centre (0, -3.5861) radius 5.1 construction
  arc A3 (-4.8429, -5.185) -> (-4.7328, -5.4862) centre (0, -3.5861) ccw projected
  dimension "d87" = 2
  dimension "d88" = 0.1
  constraints: 4 coincident, 2 centre point, 3 other
  measures "d87" radial gap between concentric circles of A1 A0
equation "\"d0\" = d_f"
equation "\"d1\" = d_b"
equation "\"d2\" = d_0"
equation "\"d3\" = d_k"
equation "\"d4\" = s_0"
equation "\"a_0_deg\" = 20deg"
equation "\"mod\" = 1"
equation "\"cp\" = 0"
equation "\"a_0\" = a_0_deg"
equation "\"x\" = -0.2"
equation "\"x_opt\" = 0.4736"
equation "\"cp_opt\" = 0.167"
equation "\"d_k2\" = 9.8"
equation "\"a_d_k2\" = 30.346816deg"
equation "\"inv_a_d_k2\" = 0.055798"
equation "\"d_02\" = 8.72862"
equation "\"a_d_02\" = 14.324785deg"
equation "\"inv_a_d_02\" = 0.005343"
equation "\"d_k3\" = 10.2"
equation "\"a_d_k3\" = 33.989448deg"
equation "\"inv_a_d_k3\" = 0.081013"
equation "\"d_k4\" = 9.4"
equation "\"a_d_k4\" = 25.88059deg"
equation "\"inv_a_d_k4\" = 0.033454"
equation "\"h_pitch\" = 104.06684"
equation "\"h_angle_deg\" = 15.2deg"
equation "\"h_angle\" = 15.2deg"
equation "\"d_f\" = 6.6"
equation "\"d_b\" = 8.457234"
equation "\"d_0\" = 9"
equation "\"d_k\" = 10.6"
equation "\"s_0\" = 1.425208"
